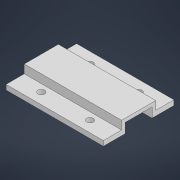
# Autodesk Inventor part: Main Carriage - Wheel Base
Saved by Autodesk Inventor 2022 (Build 260153000, 153)
## iProperties
Created: 2023-01-03
Part Number: Main Carriage - Wheel Base
Material: Generic
Document SubType Name: Modeling
Designer: Gaming
Density: 1 g/cm^3
Appearance: Default
Author: Gaming
Autodesk Inventor part; units mm, degrees
ref_plane "YZ Plane" through (0, 0, 0) normal (1, 0, 0) x (0, 1, 0)
ref_plane "XZ Plane" through (0, 0, 0) normal (0, 1, 0) x (-1, 0, 0)
ref_plane "XY Plane" through (0, 0, 0) normal (0, 0, 1) x (1, 0, 0)
sketch "Sketch1" plane through (0, 0, 0) normal (0, 1, 0) x (-1, 0, 0)
  line L0 (40, 29) -> (-40, 29)
  line L1 (-40, 29) -> (-40, 11)
  line L2 (-40, 11) -> (40, 11)
  line L3 (40, 11) -> (40, 29)
  line L4 (40, -11) -> (-40, -11)
  line L5 (-40, -11) -> (-40, -29)
  line L6 (-40, -29) -> (40, -29)
  line L7 (40, -29) -> (40, -11)
  line L8 (40, 11) -> (40, -11) construction
  point P0 (0, 0)
  point P1 (40, 0)
  point P2 (0, 29)
  dimension "d0" = 58
  dimension "d1" = 18
  dimension "d2" = 80
  constraints: 18 end point, 4 parallel, 2 equal length, 2 horizontal, 2 midpoint, 2 perpendicular, 1 horizontal alignment, 1 vertical, 1 vertical alignment
  measures "d0" distance between parallel lines of L6 L0
  measures "d1" distance of L2.end L0.start
  measures "d2" distance of L0.start L0.end
extrude "Extrusion1" add sketch "Sketch1" along normal blind 4
sketch "Sketch2" plane through (0, 4, 0) normal (0, 1, 0) x (1, 0, 0)
  line L0 (40, -29) -> (40, -11) projected
  line L1 (-40, -11) -> (40, -11)
  line L2 (40, -11) -> (40, -14)
  line L3 (40, -14) -> (-40, -14)
  line L4 (-40, -14) -> (-40, -11)
  line L5 (40, 11) -> (40, 29) projected
  line L6 (-40, 11) -> (40, 11)
  line L7 (40, 11) -> (40, 14)
  line L8 (40, 14) -> (-40, 14)
  line L9 (-40, 14) -> (-40, 11)
  point P0 (0, 0)
  dimension "d5" = 3
  dimension "d6" = 3
  constraints: 16 end point, 4 parallel, 2 horizontal, 2 perpendicular, 2 point on line
  measures "d5" distance of L1.end L2.end
  measures "d6" distance of L7.end L6.end
extrude "Extrusion2" add sketch "Sketch2" along normal blind 4
sketch "Sketch3" plane through (0, 8, 0) normal (0, 1, 0) x (1, 0, 0)
  line L0 (-40, -14) -> (40, -14) projected
  line L1 (40, 11) -> (40, 29) projected
  line L2 (-40, -14) -> (40, -14)
  line L3 (40, -14) -> (40, 14)
  line L4 (40, 14) -> (-40, 14)
  line L5 (-40, 14) -> (-40, -14)
  point P0 (0, 0)
  constraints: 8 end point, 2 parallel, 1 coincident, 1 horizontal, 1 perpendicular, 1 point on line
extrude "Extrusion3" add sketch "Sketch3" along normal blind 3
sketch "Sketch4" plane through (0, 4, 0) normal (0, 1, 0) x (1, 0, 0)
  line L0 (-40, -29) -> (40, -29) projected
  line L1 (40, 29) -> (-40, 29) projected
  line L2 (-40, 29) -> (-40, 14) projected
  line L3 (40, 14) -> (40, 29) projected
  point P0 (0, 0)
  point P1 (-20, -20)
  point P2 (20, -20)
  point P3 (-20, 20)
  point P4 (20, 20)
  dimension "d12" = 9
  dimension "d13" = 9
  dimension "d14" = 20
  dimension "d15" = 20
  constraints: 2 horizontal alignment, 2 vertical alignment
  measures "d12" distance from line of L0 point (-20, -20)
  measures "d13" distance from line of L1 point (-20, 20)
  measures "d14" distance from line of point (-20, 20) L2
  measures "d15" distance from line of point (20, 20) L3
hole "Hole1" at (-20, 4, 20) at (20, 4, 20) at (-20, 4, -20) at (20, 4, -20) direction (0, -1, 0) diameter 5.5 end through all
body "Solid1"
